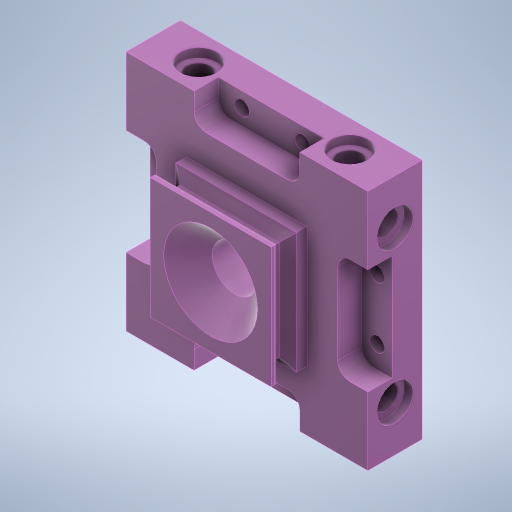
# Autodesk Inventor part: Rail-Square
Saved by Autodesk Inventor 2023.1 (Build 271208000, 208)
## iProperties
Created: 2023-06-05
Part Number: Rail-Square
Material: ABS Plastic
Document SubType Name: Modeling
Designer: hello
Density: 1.06 g/cm^3
Appearance: Smooth - Purple
Mass: 101.132 g
Surface Area: 310.671 cm^2
Volume: 95.4075 cm^3
Author: hello
Autodesk Inventor part; units mm, degrees
ref_plane "YZ Plane" through (0, 0, 0) normal (1, 0, 0) x (0, 1, 0)
ref_plane "XZ Plane" through (0, 0, 0) normal (0, 1, 0) x (-1, 0, 0)
ref_plane "XY Plane" through (0, 0, 0) normal (0, 0, 1) x (1, 0, 0)
sketch "Sketch1" plane through (0, 0, 0) normal (1, 0, 0) x (0, 1, 0)
  line L0 (-40, 0) -> (40, 0)
  line L1 (-40, 0) -> (-40, 18)
  line L2 (40, 0) -> (40, 18)
  line L3 (-40, 18) -> (40, 18)
  line L4 (0, 0) -> (0, 18) construction
  line L5 (-25, 9) -> (25, 9) construction
  circle A0 centre (-25, 9) radius 4.025
  circle A1 centre (25, 9) radius 4.025
  point P0 (0, 9)
  dimension "d0" = 80
  dimension "d9" = 18
  dimension "d10" = 50
  dimension "d11" = 8.05
  dimension "d12" = 8.05
  constraints: 12 end point, 4 coincident, 4 midpoint, 2 centre point, 2 horizontal, 2 vertical, 1 horizontal alignment, 1 parallel
  measures "d0" distance of L0.start L0.end
  measures "d9" distance of L4.start L4.end
  measures "d10" distance of L5.start L5.end
  measures "d11" diameter of A0
  measures "d12" diameter of A1
extrude "Extrusion1" add sketch "Sketch1" along normal mid plane 80
sketch "Sketch4" plane through (-40, -40, 18) normal (0, 0, 1) x (1, 0, 0)
  line L0 (0, 57.5) -> (6, 57.5)
  line L1 (10, 53.5) -> (10, 26.5)
  line L2 (6, 22.5) -> (0, 22.5)
  line L3 (0, 22.5) -> (0, 57.5)
  line L4 (0, 0) -> (0, 80) construction
  arc A0 (10, 53.5) -> (6, 57.5) centre (6, 53.5) ccw
  arc A1 (6, 22.5) -> (10, 26.5) centre (6, 26.5) ccw
  line L5 (80, 80) -> (80, 0) construction
  point P0 (40, 40)
  point P1 (10, 22.5)
  point P2 (10, 57.5)
  point P3 (0, 40)
  dimension "d24" = 10
  dimension "d25" = 35
  dimension "d26" = 4
  constraints: 8 end point, 4 point on circle, 4 point on line, 4 tangent, 2 centre point, 2 parallel, 1 equal radius, 1 horizontal, 1 midpoint, 1 perpendicular, 2 other
  measures "d24" distance of point (10, 22.5) L2.end
  measures "d25" distance of point (10, 57.5) point (10, 22.5)
  measures "d26" radius of A0
extrude "Extrusion2" cut sketch "Sketch4" against normal blind 8
sketch "Sketch5" plane through (-40, -40, 10) normal (0, 0, 1) x (1, 0, 0)
  line L0 (0, 57.5) -> (6, 57.5) projected
  line L1 (0, 22.5) -> (0, 57.5) projected
  line L2 (6, 22.5) -> (0, 22.5) projected
  arc A0 (6, 22.5) -> (10, 26.5) centre (6, 26.5) ccw projected
  line L3 (10, 53.5) -> (10, 26.5) projected
  arc A1 (10, 53.5) -> (6, 57.5) centre (6, 53.5) ccw projected
  arc A2 (74, 57.5) -> (70, 53.5) centre (74, 53.5) ccw projected
  line L4 (70, 26.5) -> (70, 53.5) projected
  arc A3 (70, 26.5) -> (74, 22.5) centre (74, 26.5) ccw projected
  line L5 (80, 57.5) -> (80, 22.5) projected
  line L6 (10, 53.5) -> (10, 26.5) projected
  line L7 (5, 50.268) -> (5, 30.268)
  line L8 (80, 22.5) -> (74, 22.5) projected
  line L9 (74, 57.5) -> (80, 57.5) projected
  point P0 (40, 40)
  point P1 (5, 40.268)
  dimension "d31" = 20
  dimension "d77" = 5
  constraints: 2 coincident, 2 end point, 1 midpoint, 1 vertical
  measures "d31" distance of L7.start L7.end
  measures "d77" distance between parallel lines of L1 L7
hole "Hole2" at (-35, 10.268, 10) at (-35, -9.732, 10) direction (0, 0, -1) diameter 5 depth 7
sketch "Sketch7" plane through (-40, 0, 0) normal (-1, 0, 0) x (0, 0, 1)
  circle A0 centre (9, 25) radius 4.025 projected
  circle A1 centre (9, -25) radius 4.025 projected
  circle A2 centre (9, 25) radius 6
  circle A3 centre (9, -25) radius 6
  point P0 (0, 0)
  dimension "d53" = 12
  dimension "d54" = 12
  constraints: 2 centre point, 2 coincident
  measures "d53" diameter of A2
  measures "d54" diameter of A3
extrude "Extrusion4" cut sketch "Sketch7" against normal blind 3
sketch "Sketch8" plane through (40, 0, 0) normal (1, 0, 0) x (0, 0, -1)
  circle A0 centre (-9, -25) radius 6 projected
  circle A1 centre (-9, 25) radius 6 projected
  point P0 (0, 0)
extrude "Extrusion5" cut sketch "Sketch8" against normal blind 3
sketch "Sketch9" plane through (-40, -40, 0) normal (0, -1, 0) x (1, 0, 0)
  line L0 (0, 0) -> (0, 18) projected
  line L1 (80, 0) -> (0, 0) projected
  line L2 (80, 18) -> (80, 0) projected
  line L3 (0, 18) -> (80, 18) projected
  line L4 (15, 9) -> (65, 9)
  point P0 (40, 0)
  point P1 (40, 9)
  point P2 (40, 18)
  point P3 (80, 9)
  dimension "d60" = 50
  constraints: 3 midpoint, 2 coincident, 2 end point, 1 horizontal, 1 horizontal alignment, 1 vertical alignment
  measures "d60" distance of L4.start L4.end
hole "Hole3" at (-25, -40, 9) at (25, -40, 9) direction (0, 1, 0) diameter 8 end through all
sketch "Sketch10" plane through (-40, -40, 0) normal (0, -1, 0) x (1, 0, 0)
  circle A0 centre (15, 9) radius 4 projected
  circle A1 centre (65, 9) radius 4 projected
  circle A2 centre (15, 9) radius 6
  circle A3 centre (65, 9) radius 6
  point P0 (40, 0)
  dimension "d68" = 12
  dimension "d69" = 12
  constraints: 2 centre point, 2 coincident
  measures "d68" diameter of A2
  measures "d69" diameter of A3
extrude "Extrusion6" cut sketch "Sketch10" against normal blind 3
sketch "Sketch11" plane through (-40, 40, 18) normal (0, 1, 0) x (1, 0, 0)
  circle A0 centre (65, 9) radius 6 projected
  circle A1 centre (15, 9) radius 6 projected
  point P0 (40, 18)
extrude "Extrusion7" cut sketch "Sketch11" against normal blind 3
pattern_circular "Circular Pattern1" count 4 over 360 about axis through (0, 0, -10) along (0, 0, 1) of "Extrusion2", "Hole2"
sketch "Sketch12" plane through (-40, 17.5, 18) normal (0, 0, 1) x (1, 0, 0)
  line L0 (20, -37.5) -> (60, -37.5)
  line L1 (60, -37.5) -> (60, 2.5)
  line L2 (60, 2.5) -> (20, 2.5)
  line L3 (20, 2.5) -> (20, -37.5)
  line L4 (20, -37.5) -> (60, 2.5) construction
  line L5 (60, -37.5) -> (20, 2.5) construction
  point P0 (40, -17.5)
  dimension "d79" = 40
  dimension "d80" = 40
  constraints: 12 end point, 2 midpoint, 2 parallel, 1 horizontal, 1 perpendicular
  measures "d79" distance of L2.end L1.end
  measures "d80" distance of L1.end L0.end
extrude "Extrusion8" add sketch "Sketch12" along normal blind 12
sketch "Sketch19" plane through (-20, -20, 18) normal (0, -1, 0) x (1, 0, 0)
  line L0 (40, 0) -> (0, 0) projected
  line L1 (40, 0) -> (40, 12) construction
  line L2 (0, 12) -> (40, 12) construction
  line L3 (0, 0) -> (0, 12) construction
  line L4 (0, 0) -> (0, 12) projected
  arc A0 (4.3, 6.7947) -> (0, 10) centre (-2.036, 2.7817) ccw
  circle A1 centre (0, 6.7947) radius 3 construction
  arc A2 (0, 3.5894) -> (4.3, 6.7947) centre (-2.036, 10.8077) ccw
  line L5 (3.5, 7.8415) -> (3.5, 5.7479)
  line L6 (0, 10) -> (0, 3.5894)
  point P0 (20, -18)
  dimension "d107" = 2
  dimension "d108" = 6
  dimension "d109" = 0
  dimension "d113" = 7.5
  dimension "d115" = 4.3
  dimension "d116" = 7.5
  dimension "d117" = 3.5
  constraints: 6 point on circle, 4 end point, 3 centre point, 2 point on line, 2 tangent, 1 collinear, 1 horizontal alignment, 1 vertical
  measures "d107" distance of L2.start L6.start
  measures "d108" diameter of A1
  measures "d109" distance from line of A1.centre L3
  measures "d113" radius of A0
  measures "d115" distance from line of A0.start L3
  measures "d116" radius of A2
  measures "d117" distance between parallel lines of L3 L5
extrude "Extrusion14" cut sketch "Sketch19" against normal through all contours L4 A0 L5 A2
pattern_circular "Circular Pattern2" count 4 over 360 about axis through (0, 0, -10) along (0, 0, 1) of "Extrusion14"
sketch "Sketch20" plane through (-40, 17.5, 30) normal (0, 0, 1) x (1, 0, 0)
  point P0 (40, -17.5)
  point P1 (40, -17.5)
  constraints: 1 coincident
hole "Hole5" at (0, 0, 30) direction (0, 0, -1) diameter 5.5 end through all counterbore diameter 15 counterbore depth 20 clearance for "Hex Head Cap Screw ISO 24017" size "M5" standard "ISO"
chamfer "Chamfer3" distance 8 angle 45 1 edges at (0, 7.5, 30)
sketch "Sketch21" plane through (40, 40, 0) normal (0, 0, -1) x (-1, 0, 0)
  line L0 (32.5, -47.5) -> (47.5, -47.5)
  line L1 (47.5, -47.5) -> (47.5, -32.5)
  line L2 (47.5, -32.5) -> (32.5, -32.5)
  line L3 (32.5, -32.5) -> (32.5, -47.5)
  line L4 (32.5, -47.5) -> (47.5, -32.5) construction
  line L5 (47.5, -47.5) -> (32.5, -32.5) construction
  line L6 (17.5, -62.5) -> (62.5, -62.5)
  line L7 (62.5, -62.5) -> (62.5, -17.5)
  line L8 (62.5, -17.5) -> (17.5, -17.5)
  line L9 (17.5, -17.5) -> (17.5, -62.5)
  point P0 (40, -40)
  dimension "d133" = 15
  dimension "d134" = 15
  dimension "d135" = 15
  constraints: 20 end point, 4 parallel, 2 midpoint, 2 perpendicular, 1 horizontal, 3 other
  measures "d133" distance of L2.end L1.end
  measures "d134" distance of L1.end L0.end
  measures "d135" distance between parallel lines of L3 L9
extrude "Extrusion15" cut sketch "Sketch21" against normal blind 5.5
chamfer "Chamfer4" distance 5.5 angle 45 8 edges at (0, -22.5, 5.5) (-22.5, 0, 5.5) (0, 7.5, 5.5) (7.5, 0, 5.5) (-7.5, 0, 5.5) (0, -7.5, 5.5) (22.5, 0, 5.5) (0, 22.5, 5.5)
fillet "Fillet4" radius 1 4 edges at (0, 20, 28) (20, 0, 28) (0, -20, 28) (-20, 0, 28)
equation "\"d12\" = d11"
equation "\"d116\" = d113"
body "Solid1"
